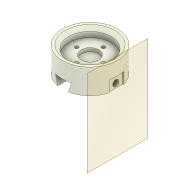
# Autodesk Inventor part: steering
Saved by Autodesk Inventor 2022 (Build 260153000, 153)
## iProperties
Created: 2024-03-23
Part Number: steering
Material: Generic
Document SubType Name: Modeling
Designer: david
Density: 1 g/cm^3
Appearance: Smooth - Ivory
Author: david
Autodesk Inventor part; units mm, degrees
ref_plane "XZ Plane" through (0, 0, 0) normal (0, 1, 0) x (-1, 0, 0)
ref_plane "XY Plane" through (0, 0, 0) normal (0, 0, 1) x (1, 0, 0)
sketch "Sketch1" plane through (0, 0, 0) normal (0, 1, 0) x (-1, 0, 0)
  circle A0 centre (0, 0) radius 10.5 construction
  circle A1 centre (0, 0) radius 15.5
  dimension "hornDia" = 21
  dimension "d1" = 5
  constraints: 2 centre point, 1 coincident
  measures "hornDia" diameter of A0
  measures "d1" radial gap between concentric circles of A1 A0
extrude "Extrusion1" add sketch "Sketch1" against normal blind 24.25
sketch "Sketch2" plane through (0, 0, 0) normal (1, 0, 0) x (0, 1, 0)
  circle A0 centre (-24.25, 0) radius 6.5 construction
  line L0 (-35.1, 0) -> (5.85, 0) construction
  line L1 (-24.25, 15.5) -> (0, 15.5) construction
  line L2 (0, 15.5) -> (0, -15.5) construction
  line L3 (0, -15.5) -> (-24.25, -15.5) construction
  line L4 (-24.25, -15.5) -> (-24.25, 15.5) construction
  circle A1 centre (-24.25, 0) radius 9.5
  line L5 (-24.25, 15.5) -> (0, 15.5) projected
  line L6 (0, 15.5) -> (0, -15.5) projected
  line L7 (0, -15.5) -> (-24.25, -15.5) projected
  line L8 (-24.25, -15.5) -> (-24.25, 15.5) projected
  point P0 (0, 0)
  point P1 (0, 0)
  dimension "shaft" = 13
  dimension "d5" = 3
  constraints: 2 centre point, 2 midpoint, 1 horizontal alignment, 1 point on line
  measures "shaft" diameter of A0
  measures "d5" radial gap between concentric circles of A1 A0
extrude "Extrusion2" add sketch "Sketch2" along normal mid plane 40 contours A1 L8 | L8 A1
sketch "Sketch4" plane through (0, 0, 0) normal (0, 1, 0) x (1, 0, 0)
  circle A0 centre (0, 0) radius 12
  circle A1 centre (0, 0) radius 15.5 projected
  dimension "d15" = 24
  constraints: 1 centre point, 1 coincident
  measures "d15" diameter of A0
sketch "Sketch3" plane through (20, -24.25, 0) normal (1, 0, 0) x (0, 0, -1)
  circle A0 centre (0, 0) radius 9.5 projected
  point P0 (0, 24.25)
  constraints: 1 coincident
hole "Hole1" at (20, -24.25, 0) direction (-1, 0, 0) diameter 13 depth 6
mirror "Mirror1" about plane through (0, 0, 0) normal (1, 0, 0) of "Hole1"
sketch "Sketch9" plane through (14, -24.25, 0) normal (1, 0, 0) x (0, 0, -1)
  circle A0 centre (0, 0) radius 6.5 projected
  point P0 (0, 24.25)
  constraints: 1 coincident
hole "Hole5" at (14, -24.25, 0) direction (-1, 0, 0) diameter 7 end through all
thicken "Thicken1" operation add thickness 0.15 both sides no extend neighbours yes toward (0, 0.0804666, -0.9967573) faces at (18, -23.727, -6.4789)
extrude "Extrusion3" add sketch "Sketch4" along normal blind 5
sketch "Sketch5" plane through (0, 0, 0) normal (1, 0, 0) x (0, 1, 0)
  arc A0 (-24.25, 9.5) -> (-24.25, -9.5) centre (-24.25, 0) ccw projected
  line L0 (-24.25, 9.5) -> (-24.25, 15.5) projected
  line L1 (-24.25, 15.5) -> (5, 15.5) projected
  line L2 (5, 15.5) -> (5, 12) projected
  line L3 (5, 12) -> (0, 12) projected
  line L4 (0, 12) -> (0, -12) projected
  line L5 (0, -12) -> (5, -12) projected
  line L6 (5, -12) -> (5, -15.5) projected
  line L7 (5, -15.5) -> (-24.25, -15.5) projected
  line L8 (-24.25, -15.5) -> (-24.25, -9.5) projected
  circle A1 centre (-24.25, 0) radius 9.5 construction
  line L9 (5, 15.5) -> (-24.25, 15.5) projected
  line L10 (-14.75, 15.5) -> (-14.75, -15.5)
  line L11 (-24.25, 15.5) -> (-24.25, 9.5) projected
  line L12 (-14.75, 15.5) -> (-24.25, 9.5)
  line L13 (-24.25, -9.5) -> (-14.75, -15.5)
  circle A2 centre (-24.25, 0) radius 3.5 projected
  point P0 (0, 0)
  constraints: 6 end point, 2 point on line, 1 coincident, 1 perpendicular, 1 vertical, 1 vertical alignment, 2 other
extrude "Extrusion4" cut sketch "Sketch5" along normal through all both and the other way through all contours L0 L1 L12 | L13 L7 L8
fillet "Fillet1" radius 5 4 edges at (13.7186, -18.0695, -7.2146) (13.7186, -18.0694, 7.2146) (-13.7186, -18.0695, -7.2146) (-13.7184, -18.0698, 7.2149)
sketch "Sketch6" plane through (0, 0, 0) normal (0, 1, 0) x (1, 0, 0)
  circle A0 centre (0, 0) radius 7.5 construction
  line L0 (-28, 0) -> (28, 0) projected
  line L1 (0, 21.7) -> (0, -21.7) projected
  point P0 (0, 7.5)
  point P1 (-7.5, 0)
  point P2 (0, -7.5)
  point P3 (7.5, 0)
  dimension "d21" = 15
  dimension "d24" = 360
  constraints: 1 coincident, 1 point on line, 1 vertical alignment, 7 other
hole "Hole2" at (0, 0, -7.5) at (-7.5, 0, 0) at (0, 0, 7.5) at (7.5, 0, 0) direction (0, -1, 0) diameter 2 depth 5 tip angle 118
sketch "Sketch7" plane through (0, 0, 0) normal (0, 1, 0) x (1, 0, 0)
  circle A0 centre (0, 0) radius 12 projected
  constraints: 1 coincident
hole "Hole3" at (0, 0, 0) direction (0, -1, 0) diameter 10 depth 2
chamfer "Chamfer1" distance 2 angle 45 1 edges at (-12, 5, 0)
chamfer "Chamfer2" distance 0.5 angle 45 2 edges at (20, -24.25, 6.65) (-20, -24.25, 6.5)
ref_plane "Work Plane1" through (0, -9, 0) normal (0, 1, 0) x (1, 0, 0)
split body "Split1" result two bodies by plane through (0, -9, 0) normal (0, 1, 0) first body at (-14.9514, -6, -1.207)
sketch "Sketch10" plane through (0, -9, 0) normal (0, 1, 0) x (1, 0, 0)
  line L0 (-3.5, -15.0997) -> (3.5, -15.0997)
  line L1 (3.5, -15.0997) -> (3.5, 15.0997)
  line L2 (3.5, 15.0997) -> (-3.5, 15.0997)
  line L3 (-3.5, 15.0997) -> (-3.5, -15.0997)
  line L4 (-3.5, -15.0997) -> (3.5, 15.0997) construction
  line L5 (3.5, -15.0997) -> (-3.5, 15.0997) construction
  line L6 (-15.0997, 3.5) -> (15.0997, 3.5)
  line L7 (15.0997, 3.5) -> (15.0997, -3.5)
  line L8 (15.0997, -3.5) -> (-15.0997, -3.5)
  line L9 (-15.0997, -3.5) -> (-15.0997, 3.5)
  line L10 (-15.0997, 3.5) -> (15.0997, -3.5) construction
  line L11 (15.0997, 3.5) -> (-15.0997, -3.5) construction
  circle A0 centre (0, 0) radius 15.5 projected
  point P0 (3.5, 3.5)
  point P1 (-3.5, 3.5)
  point P2 (-3.5, -3.5)
  point P3 (3.5, -3.5)
  dimension "d63" = 7
  dimension "d64" = 7
  constraints: 24 end point, 4 midpoint, 4 parallel, 2 horizontal, 2 perpendicular, 2 point on circle
  measures "d63" distance of L6.end L7.end
  measures "d64" distance of L1.end L2.end
extrude "Extrusion5" add sketch "Sketch10" along normal blind 5 contours L3 L8 L1 L0 | L0 A0 | L8 L9 L6 L3 | L3 L6 L1 L8 | A0 L9 | L1 L6 L7 L8 | L7 A0 | L3 L2 L1 L6 | A0 L2 bodies 3
sketch "Sketch12" plane through (0, 0, 0) normal (0, 0, 1) x (1, 0, 0)
  ellipse E0 centre (0, -39.2917) end of major axis (0, -14.75) minor radius 15.5 (11.0745, -22.1211) -> (-11.0745, -22.1211) ccw projected
  line L0 (0, 0) -> (0, -14.75)
  ellipse E1 centre (0, -39.2917) end of major axis (0, -63.8333) minor radius 15.5 (11.0745, -22.1211) -> (-11.0745, -22.1211) ccw projected
  dimension "d67" = 14.75
  constraints: 2 end point, 1 vertical, 3 other
  measures "d67" distance of L0.start L0.end
ref_plane "Work Plane2" through (0, -14.75, 0) normal (0, 1, 0) x (1, 0, 0)
sketch "Sketch18" plane through (0, 0, 0) normal (0, 0, 1) x (1, 0, 0)
  line L0 (5, 0) -> (6.5, 0) projected
  line L1 (6.5, 0) -> (6.5, -5) projected
  line L2 (6.5, -5) -> (7.5, -5.6009) projected
  line L3 (7.5, -5.6009) -> (8.5, -5) projected
  line L4 (8.5, -5) -> (8.5, 0) projected
  line L5 (8.5, 0) -> (12, 0) projected
  line L6 (12, 0) -> (12, 3) projected
  line L7 (12, 3) -> (14, 5) projected
  line L8 (14, 5) -> (15.5, 5) projected
  line L9 (15.5, 5) -> (15.5, -9) projected
  line L10 (15.5, -9) -> (-15.5, -9) projected
  line L11 (-15.5, -9) -> (-15.5, 5) projected
  line L12 (-15.5, 5) -> (-14, 5) projected
  line L13 (-14, 5) -> (-12, 3) projected
  line L14 (-12, 3) -> (-12, 0) projected
  line L15 (-12, 0) -> (-8.5, 0) projected
  line L16 (-8.5, 0) -> (-8.5, -5) projected
  line L17 (-8.5, -5) -> (-7.5, -5.6009) projected
  line L18 (-7.5, -5.6009) -> (-6.5, -5) projected
  line L19 (-6.5, -5) -> (-6.5, 0) projected
  line L20 (-6.5, 0) -> (-5, 0) projected
  line L21 (-5, 0) -> (-5, -2) projected
  line L22 (-5, -2) -> (5, -2) projected
  line L23 (5, -2) -> (5, 0) projected
  line L24 (-15.5, -9) -> (15.5, -9) projected
  line L25 (3, -9) -> (4.5, -4)
  line L26 (4.5, -4) -> (-4.5, -4)
  line L27 (-4.5, -4) -> (-3, -9)
  line L28 (3, -9) -> (-3, -9)
  line L29 (0, -48.15) -> (0, 13.8583) projected
  point P0 (0, 0)
  point P1 (3, -9)
  dimension "d97" = 6
  dimension "d98" = 9
  dimension "d99" = 5
  constraints: 8 end point, 2 point on line, 1 parallel, 1 other
  measures "d97" distance of L27.end L25.start
  measures "d98" distance of L25.end L26.end
  measures "d99" distance between parallel lines of L28 L26
extrude "Extrusion8" cut sketch "Sketch18" along normal through all both and the other way through all contours L29 L10 L27 L26 | L26 L25 L10 L29 bodies 2
ref_plane "Work Plane3" through (15.5, 0, 0) normal (1, 0, 0) x (0, 1, 0)
sketch "Sketch19" plane through (15.5, 0, 0) normal (1, 0, 0) x (0, 1, 0)
  line L0 (-9, -15.2069) -> (-9, 15.2069) projected
  line L1 (-4, -14.8324) -> (-4, 14.8324) projected
  line L2 (-4, -14.8324) -> (-4, 14.8324) projected
  line L3 (-4, 0) -> (-9, 0)
  line L4 (-9, 15.2069) -> (-9, -15.2069) projected
  point P0 (0, 0)
  point P1 (-6.5, 0)
  constraints: 3 midpoint, 2 end point
hole "Hole9" at (15.5, -6.5, 0) direction (-1, 0, 0) diameter 3.4 end through all bodies 2
sketch "Sketch22" plane through (15.5, 0, 0) normal (1, 0, 0) x (0, 1, 0)
  line L0 (-4, 14.8324) -> (-4, 15.5) projected
  line L1 (-4, 15.5) -> (-9, 15.5)
  line L2 (-10.5, 4) -> (-2.5, 4)
  line L3 (-2.5, 4) -> (-2.5, -4)
  line L4 (-2.5, -4) -> (-10.5, -4)
  line L5 (-10.5, -4) -> (-10.5, 4)
  line L6 (-10.5, 4) -> (-2.5, -4) construction
  line L7 (-2.5, 4) -> (-10.5, -4) construction
  line L8 (-9, 15.2069) -> (-9, -15.2069) projected
  point P0 (0, 0)
  point P1 (-6.5, 0)
  point P2 (-6.5, 0)
  point P3 (-9, 0)
  point P4 (-6.5, 15.5)
  point P5 (-6.5, 0)
  dimension "d117" = 8
  dimension "d118" = 8
  constraints: 14 end point, 6 midpoint, 2 horizontal, 2 parallel, 2 vertical alignment, 1 horizontal alignment, 1 perpendicular
  measures "d117" distance of L2.end L3.end
  measures "d118" distance of L3.end L4.end
extrude "Extrusion10" cut sketch "Sketch22" against normal blind 1 bodies 2
mirror "Mirror2" about plane through (0, 0, 0) normal (1, 0, 0) of "Extrusion10" bodies 2
sketch "Sketch23" plane through (-3, -9, -15.2069) normal (0, -1, 0) x (1, 0, 0)
  point P0 (3, 15.2069)
equation "\"d8\" = shaft"
equation "\"d64\" = d63"
equation "\"d118\" = d117"
equation "\"d68\" = -d67"
body "Solid2"
body "Solid3"
